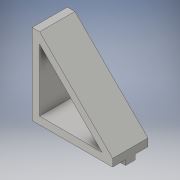
# Autodesk Inventor part: Triangle Bracket
Saved by Autodesk Inventor 2016 SP2 (Build 200236200, 236)
## iProperties
Created: 2018-01-27
Part Number: Triangle Bracket
Material: Generic
Document SubType Name: Modeling
Designer: CAD
Density: 1 g/cm^3
Appearance: Default
Author: CAD
Autodesk Inventor part; units mm, degrees
ref_plane "YZ Plane" through (0, 0, 0) normal (1, 0, 0) x (0, 1, 0)
ref_plane "XZ Plane" through (0, 0, 0) normal (0, 1, 0) x (-1, 0, 0)
ref_plane "XY Plane" through (0, 0, 0) normal (0, 0, 1) x (1, 0, 0)
sketch "Sketch1" plane through (0, 0, 0) normal (0, 0, 1) x (1, 0, 0)
  line L0 (0, 0) -> (0, 50.8)
  line L1 (0, 0) -> (50.8, 0)
  line L2 (50.8, 4.7625) -> (4.7625, 4.7625)
  line L3 (4.7625, 4.7625) -> (4.7625, 50.8)
  line L4 (50.8, 0) -> (50.8, 4.7625)
  line L5 (0, 50.8) -> (4.7625, 50.8)
  line L6 (4.7625, 50.8) -> (50.8, 4.7625)
  line L7 (4.7625, 44.0648) -> (44.0648, 4.7625)
  dimension "d0" = 50.8
  dimension "d1" = 50.8
  dimension "d2" = 4.7625
  dimension "d3" = 4.7625
  constraints: 16 end point, 2 horizontal, 2 point on line, 2 vertical, 1 parallel, 1 other
  measures "d0" distance of L0.start L0.end
  measures "d1" distance of L0.start L1.end
  measures "d2" distance between parallel lines of L1 L2
  measures "d3" distance between parallel lines of L6 L7
extrude "Extrusion1" add sketch "Sketch1" along normal blind 22.225 contours L0 L5 L3 L2 L4 L1 | L6 L2 L7 L3
sketch "Sketch2" plane through (0, 0, 0) normal (0, -1, 0) x (1, 0, 0)
  line L0 (0, 0) -> (0, 22.225) projected
  line L1 (0, 14.1605) -> (50.8, 14.1605)
  line L2 (50.8, 0) -> (50.8, 22.225) projected
  line L3 (50.8, 8.0645) -> (0, 8.0645)
  line L4 (0, 0) -> (50.8, 0) projected
  line L5 (50.8, 14.1605) -> (50.8, 8.0645)
  line L6 (0, 14.1605) -> (0, 8.0645)
  dimension "d6" = 6.096
  dimension "d7" = 8.0645
  constraints: 8 end point, 4 point on line, 1 collinear, 1 horizontal, 1 perpendicular, 1 vertical
  measures "d6" distance between parallel lines of L3 L1
  measures "d7" distance between parallel lines of L4 L3
extrude "Extrusion2" add sketch "Sketch2" along normal blind 3.175 contours L0 L1 L2 L3
body "Solid1"
